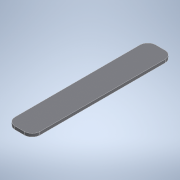
# Autodesk Inventor part: Horquilla_Elevador
Saved by Autodesk Inventor 2022.1 (Build 261234000, 234)
## iProperties
Created: 2021-09-10
Part Number: Horquilla_Elevador
Material: Genérico
Document SubType Name: Modeling
Designer: seb_0
Density: 1 g/cm^3
Appearance: Hierro - Fundido
Author: seb_0
Autodesk Inventor part; units mm, degrees
ref_plane "YZ Plane" through (0, 0, 0) normal (1, 0, 0) x (0, 1, 0)
ref_plane "XZ Plane" through (0, 0, 0) normal (0, 1, 0) x (-1, 0, 0)
ref_plane "XY Plane" through (0, 0, 0) normal (0, 0, 1) x (1, 0, 0)
sketch "Boceto1" plane through (0, 0, 0) normal (0, 1, 0) x (-1, 0, 0)
  line L0 (50, 0) -> (110, 0)
  line L1 (160, -50) -> (160, -850)
  line L2 (110, -900) -> (50, -900)
  line L3 (0, -850) -> (0, -50)
  arc A0 (160, -50) -> (110, 0) centre (110, -50) ccw
  arc A1 (50, 0) -> (0, -50) centre (50, -50) ccw
  arc A2 (110, -900) -> (160, -850) centre (110, -850) ccw
  arc A3 (0, -850) -> (50, -900) centre (50, -850) ccw
  point P0 (0, 0)
  point P1 (160, -900)
  point P2 (160, 0)
  point P3 (0, -900)
  dimension "d0" = 900
  dimension "d1" = 160
  dimension "d2" = 50
  dimension "d3" = 50
  dimension "d4" = 50
  dimension "d5" = 50
  constraints: 8 end point, 8 point on circle, 8 point on line, 8 tangent, 4 centre point, 2 parallel, 1 horizontal, 1 perpendicular
  measures "d0" distance of point (160, 0) point (160, -900)
  measures "d1" distance of point (160, -900) point (0, -900)
  measures "d2" radius of A0
  measures "d3" radius of A1
  measures "d4" radius of A2
  measures "d5" radius of A3
extrude "Extrusión1" add sketch "Boceto1" along normal blind 20
